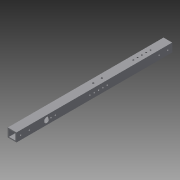
# Autodesk Inventor part: Roller Bar 18 in Segment (2)
Saved by Autodesk Inventor 2014 (Build 180170000, 170)
## iProperties
Created: 2014-02-24
Part Number: Roller Bar 18 in Segment (2)
Material: Generic
Document SubType Name: Modeling
Designer: Michael
Density: 1 g/cm^3
Appearance: Default
Author: Michael
Autodesk Inventor part; units mm, degrees
ref_plane "YZ Plane" through (0, 0, 0) normal (1, 0, 0) x (0, 1, 0)
ref_plane "XZ Plane" through (0, 0, 0) normal (0, 1, 0) x (-1, 0, 0)
ref_plane "XY Plane" through (0, 0, 0) normal (0, 0, 1) x (1, 0, 0)
sketch "Sketch1" plane through (0, 0, 0) normal (0, 0, 1) x (1, 0, 0)
  line L0 (0, 0) -> (25.4, 0)
  line L1 (25.4, 0) -> (25.4, 25.4)
  line L2 (25.4, 25.4) -> (0, 25.4)
  line L3 (0, 25.4) -> (0, 0)
  line L4 (3.175, 22.225) -> (22.225, 22.225)
  line L5 (22.225, 22.225) -> (22.225, 3.175)
  line L6 (22.225, 3.175) -> (3.175, 3.175)
  line L7 (3.175, 3.175) -> (3.175, 22.225)
  dimension "d0" = 25.4
  dimension "d1" = 25.4
  dimension "d2" = 3.175
  constraints: 16 end point, 4 parallel, 2 perpendicular, 1 horizontal, 3 other
  measures "d0" distance of L2.end L1.end
  measures "d1" distance of L1.end L0.end
  measures "d2" distance between parallel lines of L2 L4
extrude "Extrusion1" add sketch "Sketch1" along normal blind 457.2
sketch "Sketch2" plane through (25.4, 0, 0) normal (1, 0, 0) x (0, 0, -1)
  line L0 (0, 0) -> (0, 25.4) projected
  line L1 (-457.2, 0) -> (-457.2, 25.4) projected
  line L2 (0, 0) -> (-457.2, 0) projected
  circle A0 centre (-444.5, 12.7) radius 2.0701
  circle A1 centre (-419.1, 12.7) radius 2.0701
  circle A2 centre (-355.6, 12.7) radius 2.0701
  circle A3 centre (-342.9, 12.7) radius 2.0701
  circle A4 centre (-368.3, 12.7) radius 7.5406
  circle A5 centre (-241.3, 12.7) radius 2.0701
  circle A6 centre (-228.6, 12.7) radius 2.0701
  circle A7 centre (-215.9, 12.7) radius 2.0701
  circle A8 centre (-203.2, 12.7) radius 2.0701
  circle A9 centre (-190.5, 12.7) radius 2.0701
  circle A10 centre (-12.7, 12.7) radius 2.0701
  circle A11 centre (-38.1, 12.7) radius 2.0701
  dimension "d5" = 4.1402
  dimension "d6" = 12.7
  dimension "d7" = 12.7
  dimension "d10" = 25.4
  dimension "d15" = 12.7
  dimension "d16" = 63.5
  dimension "d19" = 12.7
  dimension "d24" = 15.0813
  dimension "d25" = 25.4
  dimension "d26" = 12.7
  dimension "d27" = 101.6
  dimension "d28" = 12.7
  dimension "d31" = 12.7
  dimension "d36" = 12.7
  dimension "d37" = 12.7
  dimension "d40" = 25.4
  constraints: 12 centre point, 4 horizontal, 3 equal radius, 14 other
  measures "d5" diameter of A0
  measures "d6" distance from line of L2 A0.centre
  measures "d7" distance from line of L1 A0.centre
  measures "d10" distance of A0.centre A1.centre
  measures "d15" distance from line of L2 A2.centre
  measures "d16" distance of A1.centre A2.centre
  measures "d19" distance of A2.centre A3.centre
  measures "d24" diameter of A4
  measures "d25" distance of A3.centre A4.centre
  measures "d26" distance from line of L2 A4.centre
  measures "d27" distance of A3.centre A5.centre
  measures "d28" distance from line of L2 A5.centre
  measures "d31" distance of A5.centre A6.centre
  measures "d36" distance from line of L0 A10.centre
  measures "d37" distance from line of L2 A10.centre
  measures "d40" distance of A10.centre A11.centre
extrude "Extrusion2" cut sketch "Sketch2" against normal blind 457.2
sketch "Sketch3" plane through (0, 25.4, 0) normal (0, 1, 0) x (1, 0, 0)
  line L0 (25.4, 0) -> (0, 0) projected
  line L1 (25.4, -457.2) -> (0, -457.2) projected
  line L2 (25.4, 0) -> (25.4, -457.2) projected
  circle A0 centre (12.7, -219.075) radius 2.4892
  circle A1 centre (12.7, -193.675) radius 2.4892
  circle A2 centre (12.7, -50.8) radius 2.0701
  circle A3 centre (12.7, -63.5) radius 2.0701
  circle A4 centre (12.7, -76.2) radius 2.0701
  circle A5 centre (12.7, -88.9) radius 2.0701
  circle A6 centre (12.7, -101.6) radius 2.0701
  dimension "d47" = 4.9784
  dimension "d48" = 238.125
  dimension "d49" = 12.7
  dimension "d52" = 25.4
  dimension "d57" = 4.1402
  dimension "d58" = 12.7
  dimension "d59" = 50.8
  dimension "d62" = 12.7
  constraints: 7 centre point, 2 vertical, 10 other
  measures "d47" diameter of A0
  measures "d48" distance from line of L1 A0.centre
  measures "d49" distance from line of L2 A0.centre
  measures "d52" distance of A0.centre A1.centre
  measures "d57" diameter of A2
  measures "d58" distance from line of L2 A2.centre
  measures "d59" distance from line of L0 A2.centre
  measures "d62" distance of A2.centre A3.centre
extrude "Extrusion3" cut sketch "Sketch3" against normal blind 457.2
body "Solid1"
